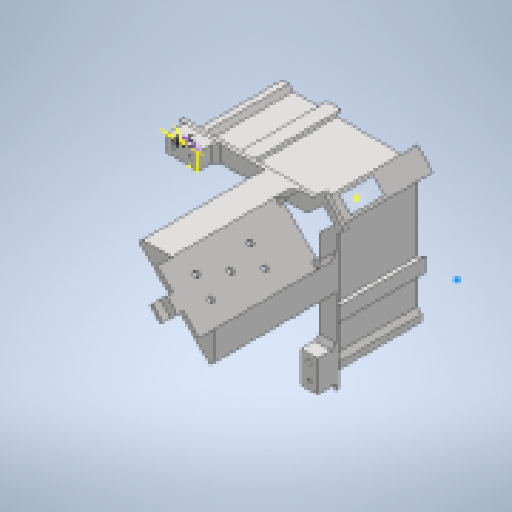
# Autodesk Inventor part: Kicker
Saved by Autodesk Inventor 2025.1 (Build 291241000, 241)
## iProperties
Created: 2025-05-21
Part Number: Kicker
Material: Generic
Document SubType Name: Modeling
Designer: User
Density: 1 g/cm^3
Appearance: Default
Author: User
## iProperties of the stored document Kicker_3DPrint.ipt
Created: 2025-06-15
Part Number: Kicker_3DPrint
Material: Generic
Document SubType Name: Modeling
Designer: User
Density: 1 g/cm^3
Appearance: Default
Author: User
Autodesk Inventor part; units mm, degrees
ref_plane "YZ Plane" through (0, 0, 0) normal (1, 0, 0) x (0, 1, 0)
ref_plane "XZ Plane" through (0, 0, 0) normal (0, 1, 0) x (-1, 0, 0)
ref_plane "XY Plane" through (0, 0, 0) normal (0, 0, 1) x (1, 0, 0)
sketch "Sketch1" plane through (0, 0, 0) normal (0, 0, 1) x (1, 0, 0)
  line L0 (-95.109205, -28.5) -> (-84.709205, -28.5)
  line L1 (-92.409205, -34) -> (-95.109205, -28.5)
  line L2 (-84.709205, -28.5) -> (-87.409205, -34)
  line L3 (-44.945496, -34) -> (-87.409205, -34)
  line L4 (-44.945496, -34) -> (-34.10235, -23.156854)
  line L5 (-34.10235, -23.156854) -> (-23.580323, -34.560198)
  line L6 (-34, -44.979875) -> (-23.580323, -34.560198)
  line L7 (-34, -87.409205) -> (-34, -44.979875)
  line L8 (-34, -87.409205) -> (-28.5, -84.709205)
  line L9 (-28.5, -84.709205) -> (-28.5, -95.109205)
  line L10 (-28.5, -95.109205) -> (-34, -92.409205)
  line L11 (-131.459205, -24.104287) -> (-125.063492, -30.5)
  line L12 (-121.263492, -34.3) -> (-91.927733, -34.3)
  line L13 (-91.927733, -34.3) -> (-94.627733, -28.8)
  line L14 (-94.627733, -28.8) -> (-85.190677, -28.8)
  line L15 (-85.190677, -28.8) -> (-87.890677, -34.3)
  line L16 (-87.890677, -34.3) -> (-44.821232, -34.3)
  line L17 (-44.821232, -34.3) -> (-34.111049, -23.589817)
  line L18 (-34.111049, -23.589817) -> (-23.996231, -34.551842)
  line L19 (-23.996231, -34.551842) -> (-34.3, -44.855611)
  line L20 (-34.3, -44.855611) -> (-34.3, -87.890677)
  line L21 (-34.3, -87.890677) -> (-28.8, -85.190677)
  line L22 (-28.8, -85.190677) -> (-28.8, -94.627733)
  line L23 (-28.8, -94.627733) -> (-34.3, -91.927733)
  line L24 (-34.3, -91.927733) -> (-34.3, -121.263492)
  line L25 (-36.8, -118.763492) -> (-36.8, -87.915465)
  line L26 (-36.8, -91.902945) -> (-36.8, -44.527184)
  line L27 (-44.492805, -36.8) -> (-91.902945, -36.8)
  line L28 (-87.915465, -36.8) -> (-118.763492, -36.8)
  line L29 (-34.3, -121.263492) -> (-36.8, -118.763492)
  line L30 (-121.263492, -34.3) -> (-118.763492, -36.8)
  line L31 (-43.992805, -36.3) -> (-34.169037, -26.476232)
  line L32 (-34.169037, -26.476232) -> (-26.768954, -34.496138)
  line L33 (-26.768954, -34.496138) -> (-36.3, -44.027184)
  line L34 (-43.992805, -36.3) -> (-44.492805, -36.8)
  line L35 (-36.3, -44.027184) -> (-36.8, -44.527184)
  point P0 (0, 0)
  dimension "d1" = 2.5
  constraints: 48 end point, 3 point on line, 1 parallel, 10 other
  measures "d1" distance between parallel lines of L12 L28
ref_plane "Work Plane1" through (-125.063492, -34, -60.437628) normal (0, 0, -1) x (0, 1, 0)
extrude "Extrusion1" add sketch "Sketch1" against normal up to surface (60.437628 mm away)
sketch "Sketch2" plane through (0, 0, 0) normal (0, 0, 1) x (1, 0, 0)
  line L0 (-91.927733, -34.3) -> (-121.263492, -34.3)
  line L1 (-94.627733, -28.8) -> (-91.927733, -34.3)
  line L2 (-85.190677, -28.8) -> (-94.627733, -28.8)
  line L3 (-87.890677, -34.3) -> (-85.190677, -28.8)
  line L4 (-44.821232, -34.3) -> (-87.890677, -34.3)
  line L5 (-34.111049, -23.589817) -> (-44.821232, -34.3)
  line L6 (-23.996231, -34.551842) -> (-34.111049, -23.589817)
  line L7 (-34.3, -44.855611) -> (-23.996231, -34.551842)
  line L8 (-34.3, -87.890677) -> (-34.3, -44.855611)
  line L9 (-28.8, -85.190677) -> (-34.3, -87.890677)
  line L10 (-28.8, -94.627733) -> (-28.8, -85.190677)
  line L11 (-34.3, -91.927733) -> (-28.8, -94.627733)
  line L12 (-34.3, -121.263492) -> (-34.3, -91.927733)
  line L13 (-31.3, -121.263492) -> (-31.3, -96.742454)
  line L14 (-31.3, -96.742454) -> (-25.8, -99.442454)
  line L15 (-25.8, -99.442454) -> (-25.8, -80.375955)
  line L16 (-25.8, -80.375955) -> (-31.3, -83.075955)
  line L17 (-31.3, -83.075955) -> (-31.3, -46.098251)
  line L18 (-31.3, -46.098251) -> (-19.837146, -34.635398)
  line L19 (-19.837146, -34.635398) -> (-34.024067, -19.260194)
  line L20 (-34.024067, -19.260194) -> (-46.063873, -31.3)
  line L21 (-46.063873, -31.3) -> (-83.075955, -31.3)
  line L22 (-83.075955, -31.3) -> (-80.375955, -25.8)
  line L23 (-80.375955, -25.8) -> (-99.442454, -25.8)
  line L24 (-99.442454, -25.8) -> (-96.742454, -31.3)
  line L25 (-96.742454, -31.3) -> (-121.263492, -31.3)
  line L26 (-131.459205, -24.104287) -> (-125.063492, -30.5)
  line L27 (-121.263492, -31.3) -> (-124.263492, -31.3)
  line L28 (-124.263492, -31.3) -> (-118.763492, -36.8)
  line L29 (-118.763492, -36.8) -> (-44.492805, -36.8)
  line L30 (-118.763492, -36.8) -> (-44.492805, -36.8)
  line L31 (-34.169037, -26.476232) -> (-26.768954, -34.496138)
  line L32 (-44.492805, -36.8) -> (-34.169037, -26.476232)
  line L33 (-34.169037, -26.476232) -> (-26.768954, -34.496138)
  line L34 (-26.768954, -34.496138) -> (-36.782811, -44.509994)
  line L35 (-36.782811, -44.509994) -> (-36.782811, -118.780681)
  line L36 (-36.782811, -118.780681) -> (-31.3, -124.263492)
  line L37 (-31.3, -124.263492) -> (-31.3, -121.263492)
  point P0 (0, 0)
  point P1 (-121.563492, -34)
  dimension "d5" = 3
  constraints: 45 end point, 3 point on line, 2 horizontal, 2 parallel, 2 perpendicular, 1 collinear, 12 other
  measures "d5" distance between parallel lines of L12 L13
extrude "Extrusion2" add sketch "Sketch2" along normal blind 2.5
sketch "Sketch3" plane through (0, 0, 0) normal (0, 0, -1) x (-1, 0, 0)
  line L0 (124.263492, -31.3) -> (121.263492, -34.3)
  line L1 (96.742454, -31.3) -> (124.263492, -31.3)
  line L2 (91.927733, -34.3) -> (121.263492, -34.3)
  line L3 (116.613744, -34) -> (120.113744, -30.5)
  line L4 (117.020851, -34.3) -> (120.020851, -31.3)
  line L5 (30.5, -120.113744) -> (34, -116.613744)
  line L6 (31.3, -120.020851) -> (34.3, -117.020851)
  line L7 (34.3, -121.263492) -> (34.3, -91.927733)
  line L8 (34.3, -121.263492) -> (31.3, -124.263492)
  line L9 (31.3, -124.263492) -> (31.3, -96.742454)
  point P0 (0, 0)
  dimension "d8" = 0.5
  dimension "d9" = 0.5
  constraints: 4 end point, 4 point on line, 2 parallel
  measures "d8" distance between parallel lines of L3 L4
  measures "d9" distance between parallel lines of L5 L6
extrude "Extrusion3" add sketch "Sketch3" along normal up to surface (60.437628 mm away)
fillet "Fillet1" radius 4 4 edges at (-118.7635, -36.8, -30.2188) (-118.7635, -36.8, 1.25) (-36.8, -118.7635, -30.2188) (-36.7828, -118.7807, 1.25)
sketch "Sketch4" plane through (0, 0, 2.5) normal (0, 0, 1) x (1, 0, 0)
  line L0 (-46.063873, -31.3) -> (-83.075955, -31.3)
  line L1 (-96.742454, -31.3) -> (-124.263492, -31.3)
  line L2 (-80.375955, -25.8) -> (-99.442454, -25.8)
  line L3 (-83.075955, -31.3) -> (-80.375955, -25.8)
  line L4 (-99.442454, -25.8) -> (-96.742454, -31.3)
  line L5 (-34.024067, -19.260194) -> (-46.063873, -31.3)
  line L6 (-124.263492, -31.3) -> (-119.935065, -35.628427)
  line L7 (-131.459205, -24.104287) -> (-125.063492, -30.5)
  line L8 (-99.442454, -25.8) -> (-129.763492, -25.8)
  line L9 (-129.763492, -25.8) -> (-124.263492, -31.3)
  line L10 (-124.263492, -31.3) -> (-96.742454, -31.3)
  line L11 (-91.927733, -34.3) -> (-117.020851, -34.3)
  line L12 (-96.742454, -31.3) -> (-99.442454, -25.8)
  line L13 (-83.075955, -31.3) -> (-80.375955, -25.8)
  line L14 (-80.375955, -25.8) -> (-99.442454, -25.8)
  line L15 (-80.375955, -25.8) -> (-40.563873, -25.8)
  line L16 (-40.563873, -25.8) -> (-46.063873, -31.3)
  line L17 (-46.063873, -31.3) -> (-83.075955, -31.3)
  line L18 (-46.063873, -31.3) -> (-83.075955, -31.3)
  line L19 (-83.075955, -31.3) -> (-80.375955, -25.8)
  line L20 (-83.075955, -31.3) -> (-80.375955, -25.8)
  line L21 (-25.8, -80.375955) -> (-31.3, -83.075955)
  line L22 (-31.3, -83.075955) -> (-31.3, -46.098251)
  line L23 (-31.3, -46.098251) -> (-19.837146, -34.635398)
  line L24 (-31.3, -96.742454) -> (-25.8, -99.442454)
  line L25 (-31.3, -124.263492) -> (-31.3, -96.742454)
  line L26 (-35.611238, -119.952254) -> (-31.3, -124.263492)
  line L27 (-30.5, -125.063492) -> (-24.104287, -131.459205)
  line L28 (-25.8, -99.442454) -> (-25.8, -129.763492)
  line L29 (-25.8, -129.763492) -> (-31.3, -124.263492)
  line L30 (-31.3, -124.263492) -> (-31.3, -96.742454)
  line L31 (-31.3, -96.742454) -> (-25.8, -99.442454)
  line L32 (-25.8, -80.375955) -> (-31.3, -83.075955)
  line L33 (-31.3, -83.075955) -> (-31.3, -46.098251)
  line L34 (-25.8, -80.375955) -> (-25.8, -40.598251)
  line L35 (-25.8, -40.598251) -> (-31.3, -46.098251)
  line L36 (-34.3, -44.855611) -> (-23.996231, -34.551842)
  line L37 (-31.3, -46.098251) -> (-31.3, -83.075955)
  line L38 (-34.3, -87.890677) -> (-34.3, -44.855611)
  line L39 (-25.8, -80.375955) -> (-31.3, -83.075955)
  point P0 (0, 0)
  constraints: 38 end point, 7 collinear, 5 parallel, 5 point on line, 2 vertical, 1 horizontal
extrude "Extrusion4" add sketch "Sketch4" against normal up to surface (2.5 mm away)
sketch "Sketch5" plane through (0, 0, 2.5) normal (0, 0, 1) x (1, 0, 0)
  line L0 (-56.270948, -42.724001) -> (-60.814958, -38.179992)
  line L1 (-56.235027, -42.759922) -> (-42.567077, -56.427872)
  line L2 (-37.987147, -61.007803) -> (-42.531156, -56.463793)
  line L3 (-37.987147, -61.007803) -> (-60.814958, -38.179992)
  line L4 (-60.814958, -38.179992) -> (-62.936278, -40.301312)
  line L5 (-62.936278, -40.301312) -> (-40.108467, -63.129123)
  line L6 (-40.108467, -63.129123) -> (-37.987147, -61.007803)
  point P0 (0, 0)
  dimension "d15" = 3
  constraints: 8 end point, 2 parallel, 1 collinear, 1 perpendicular
  measures "d15" distance of L4.end L0.end
ref_plane "Work Plane2" through (-59.602623, -59.795468, 84.008) normal (0, 0, 1) x (0.7071068, -0.7071068, 0)
extrude "Extrusion5" add sketch "Sketch5" along normal up to surface (81.508 mm away)
sketch "Sketch6" plane through (-62.936278, -40.301312, 84.008) normal (-0.7071068, -0.7071068, 0) x (-0.7071068, 0.7071068, 0)
  spline S0 degree 3 poles (-18.1417, 35.1354) (-18.1417, 35.386768) (-18.091418, 35.654735) (-17.887241, 36.147426) (-17.733358, 36.372169) (-17.37847, 36.727057) (-17.153726, 36.88094) (-16.661034, 37.085118) (-16.393066, 37.1354) (-15.890334, 37.1354) (-15.622366, 37.085118) (-15.129674, 36.88094) (-14.90493, 36.727057) (-14.550042, 36.372169) (-14.396159, 36.147426) (-14.191982, 35.654735) (-14.1417, 35.386768) (-14.1417, 34.884032) (-14.191982, 34.616065) (-14.396159, 34.123374) (-14.550042, 33.898631) (-14.90493, 33.543743) (-15.129674, 33.38986) (-15.622366, 33.185682) (-15.890334, 33.1354) (-16.393066, 33.1354) (-16.661034, 33.185682) (-17.153726, 33.38986) (-17.37847, 33.543743) (-17.733358, 33.898631) (-17.887241, 34.123374) (-18.091418, 34.616065) (-18.1417, 34.884032) (-18.1417, 35.1354) knots 0 0 0 0 0.07541033 0.07541033 0.15082067 0.15082067 0.22623054 0.22623054 0.30164041 0.30164041 0.37705028 0.37705028 0.45246015 0.45246015 0.52787048 0.52787048 0.60328081 0.60328081 0.67869115 0.67869115 0.75410148 0.75410148 0.82951135 0.82951135 0.90492122 0.90492122 0.98033109 0.98033109 1.05574096 1.05574096 1.13115129 1.13115129 1.20656163 1.20656163 1.20656163 1.20656163
  circle A0 centre (-9.2456, 17.1903) radius 2
  circle A1 centre (-23.0378, 17.1903) radius 2
  circle A2 centre (-23.0378, 53.0805) radius 2
  circle A3 centre (-9.2456, 53.0805) radius 2
  point P0 (-16.005338, 84.008)
  point P1 (-18.1417, 35.1354)
extrude "Extrusion6" cut sketch "Sketch6" against normal blind 10
sketch "Sketch7" plane through (-37.987147, -61.007803, 84.008) normal (0, 0, 1) x (0.7071068, 0.7071068, 0)
  line L0 (-40, -57.235228) -> (23.049346, 5.814118)
  line L1 (23.073655, 26.717696) -> (-40, 89.791352)
  line L2 (0, 32.2834) -> (0, 0)
  line L3 (-3, 0) -> (-3, 32.2834)
  line L4 (0, 49.791352) -> (0, -17.235228)
  line L5 (0, -17.235228) -> (-3, -17.235228)
  line L6 (-3, -17.235228) -> (-3, 49.791352)
  line L7 (-3, 49.791352) -> (0, 49.791352)
  line L8 (-3, 32.2834) -> (0, 32.2834)
  line L9 (0, 32.2834) -> (-3, 32.2834)
  line L10 (-3, 32.2834) -> (-3, 0)
  line L11 (0, 0) -> (-3, 0)
  line L12 (0, 0) -> (-3, 0)
  point P0 (70, 16.278062)
  point P1 (0, 0)
  point P2 (-3, 0)
  point P3 (-3, 32.2834)
  point P4 (0, 32.2834)
  constraints: 14 end point, 3 equal length, 3 perpendicular, 2 point on line, 1 vertical
extrude "Extrusion7" add sketch "Sketch7" against normal up to surface (81.508 mm away) contours L8 L6 L7 L4 | L4 L5 L6 L11
sketch "Sketch8" plane through (-25.8, -73.194949, 84.008) normal (0, 0, 1) x (0.7071068, 0.7071068, 0)
  arc A0 (7.142199, 21.388128) -> (31.973801, 21.388128) centre (19.558, 33.376928) ccw
  arc A1 (29.031085, 47.804128) -> (10.084915, 47.804128) centre (19.558, 33.376928) ccw
  line L0 (0, 0) -> (0, 67.02658)
  line L1 (19.558, 16.117628) -> (0, 16.117628)
  line L2 (19.558, 50.636228) -> (0, 50.636228)
  line L3 (19.558, 13.617628) -> (0, 13.617628)
  line L4 (19.558, 53.136228) -> (0, 53.136228)
  line L5 (19.558, 56.136228) -> (0, 56.136228)
  line L6 (19.558, 10.617628) -> (0, 10.617628)
  line L7 (0, 0) -> (23.049346, 23.049346)
  line L8 (23.073655, 43.952925) -> (0, 67.02658)
  line L9 (0, 67.02658) -> (0, 53.136228)
  line L10 (0, 67.02658) -> (0, 51.470231)
  line L11 (0, 67.02658) -> (13.890352, 53.136228)
  line L12 (13.617628, 13.617628) -> (0, 0)
  point P0 (70, 33.51329)
  point P1 (0, 13.617628)
  point P2 (0, 53.136228)
  dimension "d22" = 2.5
  dimension "d23" = 2.5
  dimension "d24" = 3
  dimension "d25" = 3
  constraints: 18 end point, 6 point on line, 4 parallel, 2 collinear, 2 perpendicular, 2 point on circle
  measures "d22" distance between parallel lines of L1 L3
  measures "d23" distance between parallel lines of L2 L4
  measures "d24" distance between parallel lines of L4 L5
  measures "d25" distance between parallel lines of L3 L6
extrude "Extrusion8" add sketch "Sketch8" against normal up to surface (81.508 mm away) contours L7 L6 L0 L3 | L7 L0 L6 | L4 L0 L5 L8 | L5 L0 L8
sketch "Sketch9" plane through (0, 0, 0) normal (0, 0, 1) x (1, 0, 0)
  arc A0 (-36.8, -117.106638) -> (-35.628427, -119.935065) centre (-32.8, -117.106638) ccw
  line L0 (-35.628427, -119.935065) -> (-35.611238, -119.952254)
  arc A1 (-36.782811, -117.123827) -> (-35.611238, -119.952254) centre (-32.782811, -117.123827) ccw
  line L1 (-36.782811, -117.123827) -> (-36.782811, -44.509994)
  line L2 (-36.782811, -44.509994) -> (-36.8, -44.527184)
  line L3 (-36.8, -44.527184) -> (-36.8, -117.106638)
  arc A2 (-36.8, -117.106638) -> (-35.628427, -119.935065) centre (-32.8, -117.106638) ccw
  line L4 (-35.628427, -119.935065) -> (-35.611238, -119.952254)
  arc A3 (-36.782811, -117.123827) -> (-35.611238, -119.952254) centre (-32.782811, -117.123827) ccw
  line L5 (-36.782811, -117.123827) -> (-36.782811, -44.509994)
  line L6 (-36.782811, -44.509994) -> (-36.8, -44.527184)
  line L7 (-36.8, -44.527184) -> (-36.8, -117.106638)
  point P0 (0, 0)
extrude "Extrusion9" add sketch "Sketch9" along normal up to surface (2.5 mm away)
sketch "Sketch10" plane through (-25.8, -73.194949, 84.008) normal (0.7071068, -0.7071068, 0) x (-0.7071068, -0.7071068, 0)
  circle A0 centre (18.280036, 77.110725) radius 2.6
  arc A1 (11.277671, 84.458472) -> (25.265916, 84.474147) centre (18.280036, 77.110725) ccw
  circle A2 centre (18.280036, 77.110725) radius 2.4
  circle A3 centre (18.280036, 77.110725) radius 2.5
  circle A4 centre (18.280036, 77.110725) radius 5.5
  point P0 (-70, 84.008)
  dimension "d30" = 4.8
  dimension "d31" = 5
  dimension "d32" = 3
  constraints: 3 centre point, 2 coincident
  measures "d30" diameter of A2
  measures "d31" diameter of A3
  measures "d32" radial gap between concentric circles of A3 A4
extrude "Extrusion10" add sketch "Sketch10" against normal blind 10 contours A0 | A3 | A4
sketch "Sketch11" plane through (-45.797005, -79.049819, 6.897275) normal (-0.7071068, 0.7071068, 0) x (-0.7071068, -0.7071068, 0)
  circle A0 centre (0, 0) radius 5.5 projected
  point P0 (-88.280036, -6.897275)
extrude "Extrusion11" add sketch "Sketch11" along normal blind 8.25
sketch "Sketch12" plane through (-25.8, -73.194949, 84.008) normal (0.7071068, -0.7071068, 0) x (0, 0, -1)
  arc A0 (81.508, -14.976406) -> (81.88896, -15.556349) centre (77.110725, -18.280036) ccw
  circle A1 centre (77.110725, -18.280036) radius 5.5
  point P0 (84.008, 70)
  point P1 (81.88896, -15.556349)
  point P2 (81.508, -14.976406)
extrude "Extrusion12" cut sketch "Sketch12" against normal blind 16.75
sketch "Sketch13" plane through (-51.630636, -73.216188, 6.897275) normal (-0.7071068, 0.7071068, 0) x (-0.7071068, -0.7071068, 0)
  circle A0 centre (0, 0) radius 5.5 projected
  point P0 (-88.280036, -6.897275)
extrude "Extrusion13" add sketch "Sketch13" against normal blind 4
sketch "Sketch14" plane through (-48.802209, -76.044615, 6.897275) normal (0.7071068, -0.7071068, 0) x (-0.7071068, -0.7071068, 0)
  circle A0 centre (0, 0) radius 5.5 projected
  circle A1 centre (0, 0) radius 6.5
  point P0 (-88.280036, 6.897275)
  dimension "d41" = 13
  constraints: 1 centre point, 1 coincident
  measures "d41" diameter of A1
extrude "Extrusion14" add sketch "Sketch14" against normal blind 4
sketch "Sketch15" plane through (-48.802209, -76.044615, 6.897275) normal (0.7071068, -0.7071068, 0) x (-0.7071068, -0.7071068, 0)
  circle A0 centre (0, 0) radius 6.5 projected
  circle A1 centre (0, 0) radius 4.5
  point P0 (-88.280036, 6.897275)
  dimension "d44" = 9
  constraints: 1 centre point, 1 coincident
  measures "d44" diameter of A1
extrude "Extrusion15" add sketch "Sketch15" along normal blind 4
sketch "Sketch16" plane through (-48.802209, -76.044615, 6.897275) normal (0.7071068, -0.7071068, 0) x (-0.7071068, -0.7071068, 0)
  circle A0 centre (0, 0) radius 4.5 projected
  circle A1 centre (0, 0) radius 2.35
  point P0 (-88.280036, 6.897275)
  dimension "d47" = 4.7
  constraints: 1 centre point, 1 coincident
  measures "d47" diameter of A1
extrude "Extrusion16" cut sketch "Sketch16" against normal blind 4 contours A1
ref_plane "Work Plane3" through (-73.197393, -51.649431, 6.897275) normal (-0.7071068, 0.7071068, 0) x (-0.7071068, -0.7071068, 0)
sketch "Sketch17" plane through (-73.197393, -51.649431, 6.897275) normal (-0.7071068, 0.7071068, 0) x (-0.7071068, -0.7071068, 0)
  circle A0 centre (0, 0) radius 6.5 projected
  circle A1 centre (0, 0) radius 2.35
  point P0 (-88.280036, -6.897275)
  dimension "d51" = 4.7
  constraints: 1 centre point, 1 coincident
  measures "d51" diameter of A1
extrude "Extrusion17" add sketch "Sketch17" along normal blind 8
sketch "Sketch19" plane through (-45.973782, -78.873042, 6.897275) normal (0.7071068, -0.7071068, 0) x (-0.7071068, -0.7071068, 0)
  circle A0 centre (0, 0) radius 6.5
  line L0 (-15.280036, -77.110725) -> (-15.280036, 4.397275)
  line L1 (0, -6.5) -> (-15.280036, -6.5)
  line L2 (0, 6.5) -> (-15.280036, 6.5)
  line L3 (-15.280036, -6.5) -> (-15.280036, 6.5)
  point P0 (-88.280036, 6.897275)
  point P1 (-15.280036, 4.397275)
  constraints: 6 end point, 2 perpendicular, 2 point on circle, 1 horizontal, 1 point on line, 1 tangent
extrude "Extrusion18" add sketch "Sketch19" against normal blind 8 contours A0 L1 L0 L3 L2
sketch "Sketch20" plane through (-36.8, -66.43759, 0.397275) normal (0.7071068, 0.7071068, 0) x (-0.7071068, 0.7071068, 0)
  line L0 (0, 2.102725) -> (5.693651, 2.102725)
  line L1 (0, 0) -> (0, 2.102725)
  line L2 (0, 0) -> (5.693651, 0)
  line L3 (5.693651, 2.102725) -> (5.693651, 0)
  point P0 (20.956941, -0.397275)
extrude "Extrusion19" add sketch "Sketch20" against normal up to surface surface through (-36.8, -118.763492, 0) normal (-1, 0, 0)
sketch "Sketch21" plane through (-78.854247, -45.992577, 6.897275) normal (-0.7071068, 0.7071068, 0) x (-0.7071068, -0.7071068, 0)
  circle A0 centre (0, 0) radius 6.5
  line L0 (-15.280036, 77.110725) -> (-15.280036, -4.397275)
  line L1 (0, 6.5) -> (-15.280036, 6.5)
  circle A1 centre (0, 0) radius 6.5
  line L2 (0, -6.5) -> (-15.280036, -6.5)
  line L3 (-15.280036, -6.5) -> (-15.280036, 6.5)
  point P0 (-88.280036, -6.897275)
  point P1 (-15.280036, -4.397275)
  constraints: 6 end point, 2 horizontal, 2 perpendicular, 1 point on circle, 1 point on line, 2 other
extrude "Extrusion20" add sketch "Sketch21" against normal blind 8 contours A0 L2 L3 L0 L1
sketch "Sketch22" plane through (-62.392776, -40.844814, 0.397275) normal (0.7071068, 0.7071068, 0) x (-0.7071068, 0.7071068, 0)
  line L0 (0, 2.102725) -> (5.720231, 2.102725)
  line L1 (0, 0) -> (0, 2.102725)
  line L2 (5.720231, 0) -> (0, 0)
  line L3 (5.720231, 2.102725) -> (5.720231, 0)
  point P0 (-15.23671, -0.397275)
extrude "Extrusion21" add sketch "Sketch22" along normal up to surface surface through (-44.492805, -36.8, 0) normal (0, -1, 0)
chamfer "Chamfer1" distance 15.25 angle 45 1 edges at (-65.2212, -38.0164, 13.3973)
chamfer "Chamfer2" distance 15.25 angle 45 1 edges at (-37.9976, -65.24, 13.3973)
chamfer "Chamfer3" distance 5 angle 45 4 edges at (-35.1692, -68.0684, 21.0223) (-35.1692, -68.0684, 7.9486) (-68.0496, -35.188, 7.9486) (-68.0496, -35.188, 21.0223)
sketch "Sketch24" plane through (-27.92132, -75.31627, 84.008) normal (-0.7071068, -0.7071068, 0) x (-0.7071068, 0.7071068, 0)
  line L0 (38.952925, 144.445628) -> (28.049346, 144.445628)
  line L1 (28.049346, 144.445628) -> (28.049346, 81.508)
  line L2 (38.952925, 81.508) -> (28.049346, 81.508)
  line L3 (38.952925, 144.445628) -> (38.952925, 81.508)
  line L4 (29.049346, 95.712329) -> (29.049346, 95.368555)
  line L5 (29.049346, 91.144673) -> (37.953346, 91.144673)
  line L6 (28.049346, 144.445628) -> (28.049346, 81.508)
  line L7 (38.952925, 91.144673) -> (28.049346, 91.144673)
  line L8 (28.049346, 91.144673) -> (28.049346, 113.649789)
  line L9 (28.049346, 113.649789) -> (38.952925, 113.649789)
  line L10 (38.952925, 113.649789) -> (38.952925, 91.144673)
  point P0 (33.51329, 84.008)
  point P1 (28.049346, 113.649789)
  point P2 (28.049346, 91.144673)
  point P3 (29.049346, 91.144673)
  point P4 (37.953346, 91.144673)
  dimension "d76" = 10.90358
  constraints: 10 end point, 2 horizontal, 2 parallel, 2 point on line, 1 perpendicular, 2 other
  measures "d76" distance of L8.end L9.end
extrude "Extrusion22" cut sketch "Sketch24" against normal through all contours L3 L7 L5 L1 L9
chamfer "Chamfer4" distance 2 angle 45 1 edges at (-30.469, -30.4862, -29.6418)
sketch "Sketch40" plane through (-34.169037, -26.476232, -60.437628) normal (-0.7349363, -0.6781362, 0) x (0, 0, 1)
  point P0 (60.437628, -3.712917)
sketch "Sketch41" plane through (-31.3, -124.263492, 0) normal (-0.7071068, -0.7071068, 0) x (-0.7071068, 0.7071068, 0)
  line L0 (71.17475, 31.641789) -> (60.271172, 31.641789)
  line L1 (71.17475, 60.437628) -> (71.17475, 31.641789)
  line L2 (71.17475, 60.437628) -> (60.271172, 60.437628)
  line L3 (60.271172, 60.437628) -> (60.271172, 31.641789)
  line L4 (71.17475, 31.641789) -> (60.271172, 31.641789)
  line L5 (71.17475, 60.437628) -> (71.17475, 31.641789)
  line L6 (71.17475, 60.437628) -> (60.271172, 60.437628)
  line L7 (60.271172, 60.437628) -> (60.271172, 31.641789)
  point P0 (65.735115, 0)
extrude "Extrusion36" add sketch "Sketch41" against normal up to surface surface through (-26.768954, -34.496138, 0) normal (-0.7349363, -0.6781362, 0)
sketch "Sketch43" plane through (-81.628148, -73.935343, -60.437628) normal (-0.7071068, 0.7071068, 0) x (-0.7071068, -0.7071068, 0)
  line L0 (-66.679038, 28.795839) -> (-68.680653, 30.795839)
  line L1 (-69.118935, 53.300955) -> (-69.118935, 30.795839)
  line L2 (-69.118935, 30.795839) -> (-67.11732, 28.795839)
  line L3 (-69.118935, 30.795839) -> (-67.11732, 28.795839)
  line L4 (-69.118935, 30.795839) -> (-38.301588, 0)
  line L5 (0, 0) -> (-52.517306, 0)
  line L6 (-69.118935, 30.795839) -> (-25.55183, 30.795839) construction
  line L7 (0, 28.795839) -> (-52.517306, 28.795839)
  line L8 (0, 28.795839) -> (0, 0)
  line L9 (-38.301588, 0) -> (0, 0)
  line L10 (0, 0) -> (0, 28.795839)
  line L11 (0, 28.795839) -> (-67.117538, 28.795839)
  point P0 (-110, 60.437628)
  point P1 (-52.517306, 28.795839)
  dimension "d120" = 44.98
  constraints: 12 end point, 2 perpendicular, 2 point on line, 1 collinear, 1 equal length, 1 horizontal
  measures "d120" angle of L4 L6
extrude "Extrusion37" cut sketch "Sketch43" against normal up to surface (10.903579 mm away)
sketch "Sketch44" plane through (-44.492805, -36.8, -60.437628) normal (-0.7071068, 0.7071068, 0) x (-0.7071068, -0.7071068, 0)
  line L0 (14.215718, 0) -> (0, 14.205797)
  line L1 (0, 0) -> (0, 14.205797)
  line L2 (14.215718, 0) -> (0, 0)
  point P0 (-57.482694, 60.437628)
extrude "Extrusion38" add sketch "Sketch44" along normal up to surface surface through (-44.492805, -36.8, 0) normal (0, -1, 0)
sketch "Sketch45" plane through (-36.8, -44.527184, -46.256123) normal (0.7071068, -0.7071068, 0) x (-0.7071068, -0.7071068, 0)
  line L0 (0, 0) -> (14.191409, 14.181505)
  line L1 (14.191409, 14.181505) -> (0, 14.181505)
  line L2 (0, 0) -> (0, 14.181505)
  point P0 (-57.507003, -46.256123)
extrude "Extrusion39" add sketch "Sketch45" against normal up to surface surface through (-36.8, -118.763492, 0) normal (-1, 0, 0)
sketch "Sketch47" plane through (0, 0, 2.5) normal (0, 0, 1) x (1, 0, 0)
  ellipse E0 centre (-110.440788, -31.317962) end of major axis (-111.940777, -31.312274) minor radius 1.5
  line L0 (-105.461526, -36.797108) -> (-105.420121, -25.876731)
  ellipse E1 centre (-121.440708, -31.276254) end of major axis (-122.940698, -31.270567) minor radius 1.5
  line L1 (-40.563873, -25.8) -> (-129.763492, -25.8)
  line L2 (-112.461476, -36.770567) -> (-105.461526, -36.797108)
  line L3 (-117.106638, -36.8) -> (-71.585164, -36.8)
  line L4 (-129.763492, -25.8) -> (-119.935065, -35.628427)
  line L5 (-126.41997, -25.797108) -> (-126.562265, -63.32609)
  line L6 (-105.420121, -25.876731) -> (-126.461688, -25.876731)
  line L7 (-126.461688, -25.876731) -> (-126.461688, -36.799998)
  line L8 (-126.461688, -36.799998) -> (-105.420121, -36.799998)
  line L9 (-105.420121, -36.799998) -> (-105.420121, -25.876731)
  point P0 (0, 0)
  point P1 (-73.194949, -25.8)
  point P2 (-126.420272, -25.876731)
  constraints: 8 end point, 2 parallel, 1 horizontal, 1 perpendicular, 1 point on line, 2 other
ref_plane "Work Plane4" through (-126.512975, -50.406127, 14.528338) normal (-0.0000008, -0.0002138, -1) x (0.0037916, 0.9999928, -0.0002138)
extrude "Extrusion40" add sketch "Sketch47" along normal up to surface (12.017457 mm away) contours L6 L9 L3 L8 L5
chamfer "Chamfer5" distance 2 angle 45 2 edges at (-123.1838, -32.3797, 2.5) (-118.6374, -36.4955, 2.5)
chamfer "Chamfer6" distance 2 angle 45 2 edges at (-126.4525, -34.3743, 2.5) (-124.0268, -36.8, 2.5)
sketch "Sketch48" plane through (0, 0, 2.5) normal (0, 0, 1) x (1, 0, 0)
  line L0 (-25.8, -105.030486) -> (-36.8, -105.199259)
  circle A0 centre (-31.384358, -110.116755) radius 1.5
  circle A1 centre (-31.215642, -121.11299) radius 1.5
  line L1 (-25.8, -126.030486) -> (-25.8, -105.030486)
  line L2 (-25.8, -129.763492) -> (-25.8, -73.194949)
  line L3 (-63.507444, -126.609031) -> (-25.8, -126.030486)
  line L4 (-25.8, -126.030486) -> (-36.8, -126.030486)
  line L5 (-36.8, -126.030486) -> (-36.8, -105.199259)
  line L6 (-36.8, -105.199259) -> (-25.8, -105.199259)
  line L7 (-25.8, -105.199259) -> (-25.8, -126.030486)
  point P0 (0, 0)
  constraints: 8 end point, 2 parallel, 1 horizontal, 1 perpendicular
ref_plane "Work Plane5" through (-50.831101, -126.409595, 14.5) normal (0, 0, -1) x (-0.0153412, 0.9998823, 0)
extrude "Extrusion41" add sketch "Sketch48" along normal up to surface (12 mm away) contours L6 L1 L4 L5
chamfer "Chamfer7" distance 2 angle 45 3 edges at (-32.5721, -122.9914, 2.5) (-35.6198, -119.9436, 2.5) (-36.4955, -118.6374, 2.5)
chamfer "Chamfer8" distance 2 angle 45 2 edges at (-34.5807, -126.0305, 2.5) (-36.8, -123.8112, 2.5)
chamfer "Chamfer9" distance 3 angle 45 2 edges at (-31.3, -105.1993, 2.5) (-105.4201, -31.3384, 2.5)
sketch "Sketch49" plane through (-73.194949, -25.8, 84.008) normal (0, 0, 1) x (1, 0, 0)
  line L0 (-2.12132, -2.12132) -> (45.273629, -49.51627)
  line L1 (15.9193, -24.404581) -> (22.990368, -31.475649)
  line L2 (22.990368, -31.475649) -> (27.233009, -27.233009)
  line L3 (27.233009, -27.233009) -> (20.161941, -20.161941)
  line L4 (20.161941, -20.161941) -> (15.9193, -24.404581)
  line L5 (15.9193, -24.404581) -> (27.233009, -27.233009) construction
  line L6 (22.990368, -31.475649) -> (20.161941, -20.161941) construction
  point P0 (73.194949, 25.8)
  point P1 (21.576154, -25.818795)
  dimension "d146" = 10
  constraints: 12 end point, 3 midpoint, 2 parallel, 1 perpendicular
  measures "d146" distance of L1.start L1.end
extrude "Extrusion42" add sketch "Sketch49" along normal blind 4
sketch "Sketch50" plane through (-45.961941, -53.033009, 88.008) normal (0.7071068, -0.7071068, 0) x (-0.7071068, -0.7071068, 0)
  line L0 (6, 4) -> (6, 0) projected
  line L1 (6, 4) -> (3, 4) projected
  line L2 (6, 4) -> (8.5, 4)
  line L3 (8.5, 4) -> (8.5, -5)
  line L4 (8.5, -5) -> (6, -5)
  line L5 (6, -5) -> (6, 4)
  point P0 (-70, 88.008)
  dimension "d149" = 2.5
  dimension "d150" = 9
  constraints: 8 end point, 2 parallel, 1 horizontal, 1 perpendicular
  measures "d149" distance of L3.end L4.end
  measures "d150" distance of L2.end L3.end
extrude "Extrusion43" add sketch "Sketch50" against normal up to surface (10 mm away)
chamfer "Chamfer10" distance 5.5 angle 45 1 edges at (-51.6188, -51.6188, 84.008)
chamfer "Chamfer11" distance 3 angle 45 4 edges at (-30.6146, -58.7513, 2.5) (-37.0669, -61.928, 2.5) (-61.8222, -37.1727, 2.5) (-58.462, -30.711, 2.5)
chamfer "Chamfer12" distance 5 angle 45 2 edges at (-64.9666, -36.8, 0.3973) (-36.8, -64.9948, 0.3973)
sketch "Sketch54" plane through (-126.420272, -25.876731, 14.523093) normal (0, 1, 0) x (1, 0, -0.0000008)
  line L0 (21.000151, 0) -> (0, 0)
  line L1 (21.000158, 9.023076) -> (21.000151, 0)
  line L2 (24.000161, 12.023073) -> (21.000158, 9.023076)
  line L3 (0.00001, 12.023093) -> (24.000161, 12.023073)
  line L4 (0.00001, 12.023093) -> (0, 0)
  point P0 (126.420283, 14.52299)
extrude "Extrusion44" add sketch "Sketch54" along normal up to surface (0.076731 mm away)
sketch "Sketch55" plane through (-126.420272, -25.8, 14.523093) normal (0.0000008, 0, 1) x (1, 0, -0.0000008)
  line L0 (21.000151, 0) -> (0, 0)
  line L1 (12.066637, 0.5) -> (5.763956, 6.802681)
  line L2 (-3.843265, 0.5) -> (12.066637, 0.5)
  line L3 (12.066637, 0.5) -> (13.566637, 0.5)
  line L4 (13.566637, 0.5) -> (10.354309, 3.651341)
  line L5 (13.566637, 0.5) -> (14.076314, 0)
  line L6 (14.076314, 0) -> (21.000151, 0)
  line L7 (21.000151, -0.076731) -> (0, -0.076731)
  line L8 (21.000151, 0) -> (16.658149, 3.651341)
  line L9 (16.658149, 3.651341) -> (10.354309, 3.651341)
  point P0 (126.420283, 25.8)
  dimension "d168" = 1.5
  dimension "d169" = 4.5
  constraints: 12 end point, 3 point on line, 1 horizontal, 1 parallel
  measures "d168" distance of L1.start L3.end
  measures "d169" distance of L3.end L4.end
extrude "Extrusion45" add sketch "Sketch55" against normal up to surface (12.023093 mm away)
sketch "Sketch56" plane through (0, 0, 2.5) normal (0, 0, 1) x (1, 0, 0)
  line L0 (-19.436039, -120.21755) -> (-25.8, -113.853589)
  line L1 (-25.8, -113.853589) -> (-25.8, -129.763492)
  line L2 (-25.8, -113.853589) -> (-25.8, -112.353589)
  line L3 (-25.8, -40.598251) -> (-25.8, -129.763492)
  line L4 (-25.8, -112.353589) -> (-22.618019, -115.53557)
  line L5 (-25.8, -105.199259) -> (-36.8, -105.199259)
  line L6 (-25.8, -105.199259) -> (-22.618019, -108.381239)
  line L7 (-25.8, -105.199259) -> (-21.3, -105.199259) construction
  line L8 (-22.618019, -108.381239) -> (-22.618019, -115.53557)
  line L9 (-25.8, -105.199259) -> (-25.8, -112.353589)
  point P0 (0, 0)
  dimension "d172" = 1.5
  dimension "d173" = 4.5
  dimension "d174" = 45
  constraints: 12 end point, 1 equal length, 1 horizontal, 1 point on line, 1 vertical
  measures "d172" distance of L0.end L2.end
  measures "d173" distance of L2.end L4.end
  measures "d174" angle of L6 L7
extrude "Extrusion46" add sketch "Sketch56" along normal up to surface (12 mm away)
body "Solid1"
